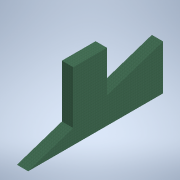
# Autodesk Inventor part: roof
Saved by Autodesk Inventor 2020.2 (Build 242310000, 310)
## iProperties
Created: 2020-03-27
Part Number: roof
Material: Generic
Document SubType Name: Modeling
Designer: robst
Density: 1 g/cm^3
Appearance: Green Polished
Author: robst
Autodesk Inventor part; units mm, degrees
ref_plane "YZ Plane" through (0, 0, 0) normal (1, 0, 0) x (0, 1, 0)
ref_plane "XZ Plane" through (0, 0, 0) normal (0, 1, 0) x (-1, 0, 0)
ref_plane "XY Plane" through (0, 0, 0) normal (0, 0, 1) x (1, 0, 0)
sketch "Sketch1" plane through (0, 0, 0) normal (1, 0, 0) x (0, 1, 0)
  line L0 (0, 0) -> (1219.2, 0)
  line L1 (1219.2, 0) -> (0, 3657.6)
  line L2 (0, 3657.6) -> (0, 0)
  dimension "rise" = 1219.2
  dimension "run" = 3657.6
  dimension "roofAngle" = 18.435
  constraints: 6 end point, 1 horizontal, 1 vertical
  measures "rise" distance of L0.start L0.end
  measures "run" distance of L1.end L0.start
  measures "roofAngle" angle of L1 L2
extrude "Extrusion1" add sketch "Sketch1" along normal mid plane 304.8
sketch "Sketch2" plane through (152.4, 0, 0) normal (1, 0, 0) x (0, 0, -1)
  line L0 (0, 1219.2) -> (-3657.6, 0) projected
  line L1 (-2438.4, 406.4) -> (-2438.4, 1833.2707)
  line L2 (-2438.4, 1833.2707) -> (-1524, 1833.2707)
  line L3 (-1524, 1833.2707) -> (-1524, 711.2)
  point P0 (0, 0)
  dimension "d5" = 1219.2
  dimension "d6" = 914.4
  constraints: 6 end point, 2 perpendicular, 2 point on line, 1 vertical
  measures "d5" distance from line of L0.end L1
  measures "d6" distance of L1.end L2.end
extrude "Extrusion2" add sketch "Sketch2" against normal blind 304.8
body "Solid1"
